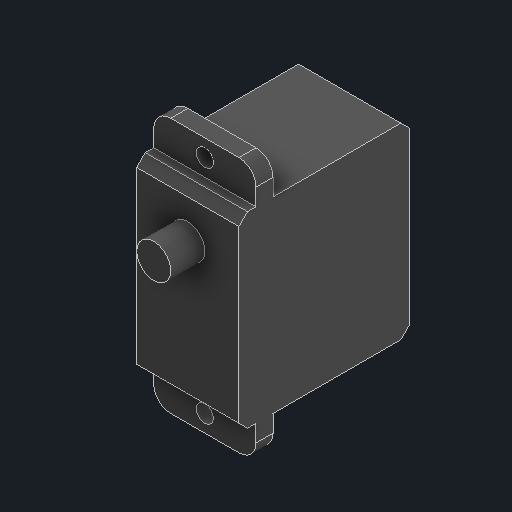
# Autodesk Inventor part: servo
Saved by Autodesk Inventor 2023 (Build 270158030, 158C)
## iProperties
Created: 2022-03-29
Part Number: servo
Material: Generic
Document SubType Name: Modeling
Designer: kardo
Density: 1 g/cm^3
Appearance: Dark Plastic
Author: kardo
Autodesk Inventor part; units mm, degrees
ref_plane "YZ Plane" through (0, 0, 0) normal (1, 0, 0) x (0, 1, 0)
ref_plane "XZ Plane" through (0, 0, 0) normal (0, 1, 0) x (-1, 0, 0)
ref_plane "XY Plane" through (0, 0, 0) normal (0, 0, 1) x (1, 0, 0)
derived "parameters_powertrain.ipt"
sketch "sk_profile" plane through (0, 0, 0) normal (1, 0, 0) x (0, 1, 0)
  line L0 (0, 28.8) -> (0, -4.8) construction
  line L1 (-21, 0) -> (21, 0) construction
  line L2 (-11, 20) -> (11, 20)
  line L3 (11, 20) -> (11, 18)
  line L4 (11, 18) -> (15, 18)
  line L5 (-11, 20) -> (-11, 18)
  line L6 (-11, 18) -> (-15, 18)
  line L7 (-15, 18) -> (-15, 16)
  line L8 (-15, 16) -> (-11, 16)
  line L9 (-11, 16) -> (-11, 0)
  line L10 (15, 18) -> (15, 16)
  line L11 (15, 16) -> (11, 16)
  line L12 (11, 16) -> (11, 0)
  line L13 (-11, 0) -> (11, 0)
  line L14 (5.5, 20) -> (5.5, 24) construction
  point P0 (0, 0)
  dimension "d2" = 22
  dimension "d3" = 24
  dimension "d4" = 4
  dimension "d5" = 4
  dimension "d6" = 16
  dimension "d7" = 2
  dimension "d8" = 5.5
  constraints: 26 end point, 9 parallel, 5 collinear, 4 point on line, 1 coincident, 1 other
  measures "d2" distance between parallel lines of L12 L9
  measures "d3" distance from line of L1 L14.end
  measures "d4" distance of L14.start L14.end
  measures "d5" distance of L5.end L6.end
  measures "d6" distance between parallel lines of L13 L8
  measures "d7" distance of L6.end L7.end
  measures "d8" distance between parallel lines of L14 L0
extrude "depth" add sketch "sk_profile" along normal mid plane 12
sketch "sk_shaft" plane through (-6, -11, 20) normal (0, 0, 1) x (1, 0, 0)
  circle A0 centre (6, 16.5) radius 2
  point P0 (6, 11)
  dimension "d25" = 4
  constraints: 1 centre point, 1 coincident
  measures "d25" diameter of A0
extrude "shaft" add sketch "sk_shaft" along normal up to surface (4 mm away)
chamfer "chamfer_top" distance 1 angle 45 2 edges at (0, 11, 20) (0, -11, 20)
chamfer "chamfer_bottom" distance 1 angle 45 2 edges at (0, 11, 0) (0, -11, 0)
sketch "sk_drill" plane through (0, 0, 0) normal (0, 0, 1) x (1, 0, 0)
  line L0 (0, -18.2) -> (0, 18.2) construction
  line L1 (-18.2, 0) -> (18.2, 0) construction
  line L2 (0, -13) -> (0, 13) construction
  point P0 (0, 0)
  point P1 (0, 0)
  dimension "d17" = 26
  constraints: 2 coincident, 2 end point, 2 midpoint, 2 point on line
  measures "d17" distance of point (0, 13) point (0, -13)
hole "drill_pad" at (0, -13, 0) at (0, 13, 0) direction (0, 0, 1) diameter 2 end through all both
fillet "round_pads" radius 2 4 edges at (6, 15, 17) (-6, 15, 17) (6, -15, 17) (-6, -15, 17)
equation "\"d2\" = servo_width"
equation "\"d3\" = servo_height"
equation "\"d5\" = servo_pad_width"
equation "\"d6\" = servo_pad_height"
equation "\"d8\" = servo_shaft_offset"
equation "\"d9\" = servo_depth"
equation "\"d17\" = servo_width + 2 * servo_pad_drill_outset"
equation "\"d18\" = servo_pad_drill_diam"
equation "\"servo_width\" = 22"
equation "\"servo_height\" = 24"
equation "\"servo_pad_width\" = 4"
equation "\"servo_pad_height\" = 16"
equation "\"servo_shaft_offset\" = 5.5"
equation "\"servo_depth\" = 12"
equation "\"servo_pad_drill_diam\" = 2"
equation "\"servo_pad_drill_outset\" = 2"
body "Solid1"
